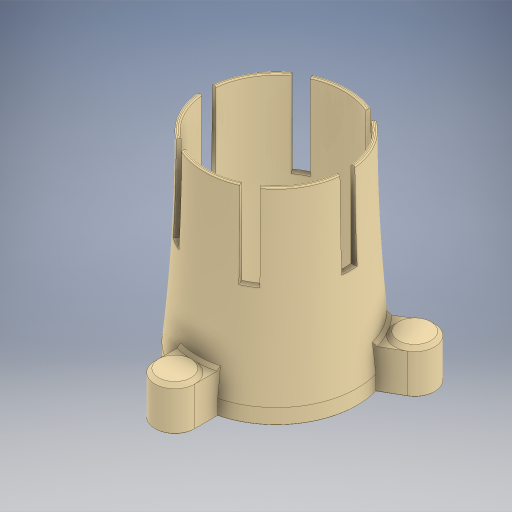
# Autodesk Inventor part: capacitor_cup
Saved by Autodesk Inventor 2023 (Build 270158000, 158)
## iProperties
Created: 2024-12-20
Part Number: capacitor_cup
Material: Типовые
Document SubType Name: Modeling
Designer: Ivan
Density: 1 g/cm^3
Appearance: Пшеничный
Mass: 3.39616 g
Surface Area: 55.8883 cm^2
Volume: 3.39616 cm^3
Author: Ivan
Autodesk Inventor part; units mm, degrees
ref_plane "YZ Plane" through (0, 0, 0) normal (1, 0, 0) x (0, 1, 0)
ref_plane "XZ Plane" through (0, 0, 0) normal (0, 1, 0) x (-1, 0, 0)
ref_plane "XY Plane" through (0, 0, 0) normal (0, 0, 1) x (1, 0, 0)
sketch "Эскиз1" plane through (0, 0, 0) normal (0, 1, 0) x (-1, 0, 0)
  circle A0 centre (0, 0) radius 11.1
  circle A1 centre (0, 0) radius 11.7
  dimension "d0" = 22.2
  dimension "d1" = 0.6
  constraints: 2 centre point, 2 coincident
  measures "d0" diameter of A0
  measures "d1" radial gap between concentric circles of A1 A0
sketch "Эскиз2" plane through (0, 0, 0) normal (1, 0, 0) x (0, 1, 0)
  line L0 (0, -11.7) -> (0, 11.7) projected
  line L1 (0, 11.7) -> (-30, 11.7) construction
  line L2 (0, -11.7) -> (-30, -11.7) construction
  line L3 (0, -11.1) -> (0, 11.1) projected
  line L4 (0, 11.1) -> (-30, 11.1)
  line L5 (0, -11.1) -> (-30, -11.1)
  line L6 (-30, 11.7) -> (-30, -11.7) construction
  line L7 (-30, 11.7) -> (-30, 13.2) construction
  line L8 (-30, -11.7) -> (-30, -13.2) construction
  arc A0 (-30, 13.2) -> (0, 11.7) centre (0, 312.45) ccw
  arc A1 (0, -11.7) -> (-30, -13.2) centre (0, -312.45) ccw
  line L9 (0, 0) -> (-30, 0)
  line L10 (-30, 13.2) -> (-32.5, 13.2)
  line L11 (-32.5, 13.2) -> (-32.5, -13.2)
  line L12 (-32.5, -13.2) -> (-30, -13.2)
  line L13 (-30, -13.2) -> (-30, 13.2) construction
  line L14 (-30, 11.1) -> (-30, -11.1)
  line L15 (-30, 0) -> (-32.5, 0)
  point P0 (-30, 0)
  dimension "d2" = 1.5
  dimension "d3" = 30
  dimension "d5" = 2.5
  constraints: 28 end point, 4 equal length, 4 horizontal, 4 point on circle, 2 centre point, 2 midpoint, 2 parallel, 2 point on line, 2 tangent, 2 vertical, 1 collinear, 1 perpendicular
  measures "d2" distance of L1.end L7.end
  measures "d3" distance of L0.start L2.end
  measures "d5" distance of L11.end L12.end
revolve "Вращение2" add sketch "Эскиз2" angle 360 about axis through (0, 0, 0) along (0, -1, 0) contours L4 L14 L15 L11 L10 A0 L0
sketch "Эскиз3" plane through (0, 0, 0) normal (0, 1, 0) x (1, 0, 0)
  line L0 (18.48, 0) -> (-18.48, 0)
  circle A0 centre (0, 0) radius 11.1
  line L1 (-11.039193, -1.160266) -> (-13.077911, -1.374544)
  line L2 (-11.039193, 1.160266) -> (-13.077911, 1.374544)
  line L3 (-11.1, 0) -> (-9.050052, 0) construction
  line L4 (-6.524416, -8.980089) -> (-7.729345, -10.638531)
  line L5 (-4.514777, -10.140355) -> (-5.348566, -12.013075)
  line L6 (4.514777, -10.140355) -> (5.348566, -12.013075)
  line L7 (6.524416, -8.980089) -> (7.729345, -10.638531)
  line L8 (11.039193, -1.160266) -> (13.077911, -1.374544)
  line L9 (11.039193, 1.160266) -> (13.077911, 1.374544)
  line L10 (6.524416, 8.980089) -> (7.729345, 10.638531)
  line L11 (4.514777, 10.140355) -> (5.348566, 12.013075)
  line L12 (-4.514777, 10.140355) -> (-5.348566, 12.013075)
  line L13 (-6.524416, 8.980089) -> (-7.729345, 10.638531)
  circle A1 centre (0, 0) radius 13.149948
  point P0 (7.729345, -10.638531)
  point P1 (6.524416, -8.980089)
  point P2 (4.514777, -10.140355)
  point P3 (11.039193, 1.160266)
  point P4 (11.039193, -1.160266)
  point P5 (13.077911, -1.374544)
  point P6 (7.729345, 10.638531)
  point P7 (5.348566, 12.013075)
  point P8 (4.514777, 10.140355)
  point P9 (6.524416, 8.980089)
  point P10 (-5.348566, 12.013075)
  point P11 (-7.729345, 10.638531)
  point P12 (-6.524416, 8.980089)
  point P13 (-13.077911, -1.374544)
  point P14 (-5.348566, -12.013075)
  point P15 (-4.514777, -10.140355)
  dimension "d8" = 12
  dimension "d9" = 6
  dimension "d12" = 360
  constraints: 26 end point, 13 point on line, 3 coincident, 3 point on circle, 2 equal length, 1 collinear, 44 other
  measures "d8" angle of L1 L2
  measures "d9" angle of L3 L1
extrude "Выдавливание1" cut sketch "Эскиз3" against normal blind 14 contours A1 L8 A0 L0 | L0 A0 L9 A1 | A0 L1 A1 L0 | L0 A1 L2 A0 | L10 A0 L11 A1 | A1 L6 A0 L7 | L13 A1 L12 A0 | A0 L5 A1 L4
fillet "Сопряжение1" radius 0.2 14 edges at (-9.6129, 0, 5.55) (2.3078, 0, 10.8574) (-2.3078, 0, 10.8574) (-9.6129, 0, -5.55) (0, 0, -11.1) (9.6129, 0, -5.55) (9.6129, 0, 5.55) (10.1325, 0, 5.85) (10.1325, 0, -5.85) (0, 0, -11.7) (-10.1325, 0, -5.85) (-10.1325, 0, 5.85) (2.4326, 0, 11.4443) (-2.4326, 0, 11.4443)
sketch "Эскиз4" plane through (0, -32.5, 0) normal (0, -1, 0) x (1, 0, 0)
  circle A0 centre (0, 0) radius 10.8 projected
  circle A1 centre (0, 0) radius 10
  dimension "d18" = 20
  constraints: 1 centre point, 1 coincident
  measures "d18" diameter of A1
extrude "Выдавливание2" cut sketch "Эскиз4" against normal blind 14 contours A1
sketch "Эскиз5" plane through (0, -32.5, 0) normal (0, -1, 0) x (1, 0, 0)
  circle A0 centre (0, 0) radius 10
  circle A1 centre (0, 0) radius 13.2
  circle A2 centre (0, 0) radius 13.2
  circle A3 centre (0, 0) radius 10
  circle A4 centre (0, 16.55) radius 2
  line L0 (0, 26.4) -> (0, -19.8) construction
  circle A5 centre (0, 16.55) radius 3.25
  line L1 (-3.25, 16.55) -> (3.25, 16.55) construction
  line L2 (-3.25, 16.55) -> (-3.25, 12.793651)
  line L3 (3.25, 16.55) -> (3.25, 12.793651)
  circle A6 centre (-14.33272, -8.275) radius 3.25
  circle A7 centre (-14.33272, -8.275) radius 2
  line L4 (-12.70772, -11.089583) -> (-9.454627, -9.211408)
  line L5 (-15.95772, -5.460417) -> (-12.704627, -3.582243)
  circle A8 centre (14.33272, -8.275) radius 3.25
  circle A9 centre (14.33272, -8.275) radius 2
  line L6 (15.95772, -5.460417) -> (12.704627, -3.582243)
  line L7 (12.70772, -11.089583) -> (9.454627, -9.211408)
  point P0 (0, 13.2)
  point P1 (0, 13.3)
  point P2 (-11.518138, -6.65)
  point P3 (11.518138, -6.65)
  dimension "d23" = 4
  dimension "d25" = 6.5
  dimension "d26" = 0.1
  dimension "d29" = 360
  constraints: 14 end point, 11 point on circle, 6 centre point, 3 coincident, 3 point on line, 2 vertical, 1 horizontal, 1 midpoint, 36 other
  measures "d23" diameter of A4
  measures "d25" diameter of A5
  measures "d26" distance of point (0, 13.2) point (0, 13.3)
extrude "Выдавливание3" add sketch "Эскиз5" against normal blind 2.5 contours A1 L2 A5 L3 | L6 A8 L7 A1 | A5 | A8 | A1 L4 A6 L5 | A6
sketch "Эскиз7" plane through (0, -30, 0) normal (0, 1, 0) x (1, 0, 0)
  circle A0 centre (-14.33272, 8.275) radius 3.25
  circle A1 centre (0, -16.55) radius 3.25
  circle A2 centre (14.33272, 8.275) radius 3.25
  circle A3 centre (14.33272, 8.275) radius 2
  circle A4 centre (-14.33272, 8.275) radius 2
  circle A5 centre (0, -16.55) radius 2
  point P0 (0, 0)
extrude "Выдавливание4" add sketch "Эскиз7" along normal blind 4.5
sketch "Эскиз8" plane through (0, -25.5, 16.55) normal (0, 1, 0) x (1, 0, 0)
  circle A0 centre (0, 0) radius 2
  circle A1 centre (14.33272, 24.825) radius 2
  circle A2 centre (-14.33272, 24.825) radius 2
  point P0 (0, 16.55)
extrude "Выдавливание5" add sketch "Эскиз8" against normal blind 1.5
chamfer "Фаска1" distance 0.6 angle 45 3 edges at (-3.25, -25.5, 16.55) (11.0827, -25.5, -8.275) (-17.5827, -25.5, -8.275)
chamfer "Фаска2" distance 0.1 angle 45 13 edges at (3.25, -32.5, 14.6718) (0, -32.5, 19.8) (-3.25, -32.5, 14.6718) (11.4315, -32.5, 6.6) (14.3312, -32.5, -4.5213) (17.1473, -32.5, -9.9) (11.0812, -32.5, -10.1505) (0, -32.5, -13.2) (-11.0812, -32.5, -10.1505) (-17.1473, -32.5, -9.9) (-14.3312, -32.5, -4.5213) (-11.4315, -32.5, 6.6) (-10, -32.5, 0)
sketch "Эскиз10" plane through (0, -30, 0) normal (0, 1, 0) x (1, 0, 0)
  arc A0 (3.25, -16.55) -> (-3.25, -16.55) centre (0, -16.55) ccw
  line L0 (3.25, -16.55) -> (3.25, -12.793651)
  arc A1 (-3.25, -12.793651) -> (3.25, -12.793651) centre (0, 0) ccw
  line L1 (-3.25, -12.793651) -> (-3.25, -16.55)
  arc A2 (-15.95772, 5.460417) -> (-12.70772, 11.089583) centre (-14.33272, 8.275) ccw
  line L2 (-15.95772, 5.460417) -> (-12.704627, 3.582243)
  arc A3 (-9.454627, 9.211408) -> (-12.704627, 3.582243) centre (0, 0) ccw
  line L3 (-9.454627, 9.211408) -> (-12.70772, 11.089583)
  arc A4 (12.70772, 11.089583) -> (15.95772, 5.460417) centre (14.33272, 8.275) ccw
  line L4 (12.70772, 11.089583) -> (9.454627, 9.211408)
  arc A5 (12.704627, 3.582243) -> (9.454627, 9.211408) centre (0, 0) ccw
  line L5 (12.704627, 3.582243) -> (15.95772, 5.460417)
ref_plane "РабПлоскость1" through (-14.33272, -26.1, -8.275) normal (0, 1, 0) x (1, 0, 0)
extrude "Выдавливание6" add sketch "Эскиз10" along normal up to surface (3.9 mm away)
sketch "Эскиз12" plane through (-14.33272, -26.1, -8.275) normal (0, 1, 0) x (0.8660254, 0, 0.5)
  arc A0 (3.756349, 3.25) -> (3.756349, -3.25) centre (16.55, 0) ccw
  arc A1 (20.132243, -12.704627) -> (25.761408, -9.454627) centre (16.55, 0) ccw
  arc A2 (25.761408, 9.454627) -> (20.132243, 12.704627) centre (16.55, 0) ccw
  circle A3 centre (16.55, 0) radius 12.792713
  line L0 (0, 3.25) -> (3.756349, 3.25)
  line L1 (3.756349, 3.25) -> (4.177005, 3.25)
  line L2 (3.756349, -3.25) -> (0, -3.25)
  line L3 (3.756349, -3.25) -> (4.177005, -3.25)
  arc A4 (3.756349, -3.25) -> (20.132243, -12.704627) centre (16.55, 0) ccw
  line L4 (20.132243, -12.704627) -> (19.921915, -12.340328)
  line L5 (22.010417, -15.95772) -> (20.132243, -12.704627)
  line L6 (25.761408, -9.454627) -> (25.55108, -9.090328)
  line L7 (25.761408, -9.454627) -> (27.639583, -12.70772)
  line L8 (25.761408, 9.454627) -> (25.55108, 9.090328)
  line L9 (20.132243, 12.704627) -> (19.921915, 12.340328)
  line L10 (20.132243, 12.704627) -> (22.010417, 15.95772)
  dimension "d47" = 25.58543
  constraints: 12 end point, 6 point on circle, 5 collinear, 1 centre point, 1 coincident, 1 parallel
  measures "d47" diameter of A3
extrude "Выдавливание7" add sketch "Эскиз12" against normal up to surface (3.9 mm away) contours L1 A3 L3 A0 | L4 A3 L6 A1 | L9 A2 L8 A3
chamfer "Фаска3" distance 0.5 angle 45 4 edges at (-1.6384, -26.1, 12.7297) (1.6384, -26.1, 12.7297) (-11.1151, -26.1, -6.4173) (11.1151, -26.1, -6.4173)
equation "\"d9\" = 0.5 * d8"
